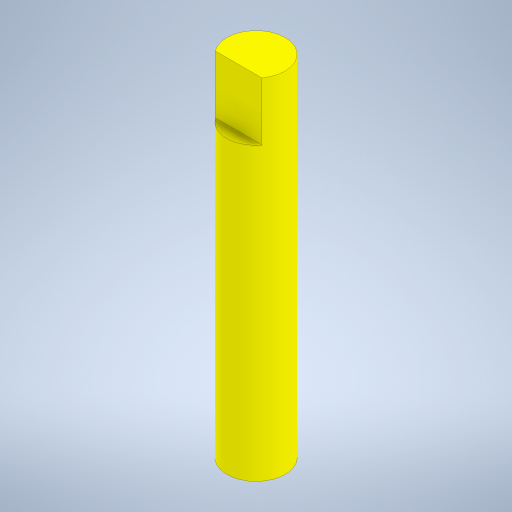
# Autodesk Inventor part: 팔
Saved by Autodesk Inventor 2023 (Build 270158000, 158)
## iProperties
Created: 2022-10-29
Part Number: 팔
Material: 일반
Document SubType Name: Modeling
Designer: 전상현
Density: 1 g/cm^3
Appearance: 기본값(2)
Author: 전상현
Autodesk Inventor part; units mm, degrees
ref_plane "YZ Plane" through (0, 0, 0) normal (1, 0, 0) x (0, 1, 0)
ref_plane "XZ Plane" through (0, 0, 0) normal (0, 1, 0) x (-1, 0, 0)
ref_plane "XY Plane" through (0, 0, 0) normal (0, 0, 1) x (1, 0, 0)
sketch "스케치1" plane through (0, 0, 0) normal (0, 1, 0) x (-1, 0, 0)
  circle A0 centre (0, 0) radius 2.5
  dimension "d0" = 5
  constraints: 1 centre point, 1 coincident
  measures "d0" diameter of A0
extrude "돌출1" add sketch "스케치1" along normal blind 30
sketch "스케치2" plane through (0, 30, 0) normal (0, 1, 0) x (1, 0, 0)
  circle A0 centre (0, 0) radius 2.5 projected
  line L0 (-2, -1.5) -> (2, -1.5)
  dimension "d3" = 1.5
  constraints: 2 end point, 2 point on circle, 1 horizontal
  measures "d3" distance from line of L0 A0.centre
extrude "돌출2" cut sketch "스케치2" against normal blind 5 contours L0 A0 picked at (-0.534, -1.6398)
